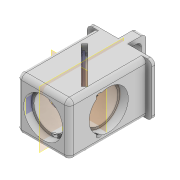
# Autodesk Inventor part: 30_Cube_Insert_Filter_Revolver_Filter_base_single_v3
Saved by Autodesk Inventor 2022 (Build 260153000, 153)
## iProperties
Created: 2021-11-01
Part Number: 30_Cube_Insert_Filter_Revolver_Filter_base_single_v3
Material: Generic
Document SubType Name: Modeling
Designer: diederichbenedict
Density: 1 g/cm^3
Appearance: Default
Author: diederichbenedict
Autodesk Inventor part; units mm, degrees
ref_plane "YZ Plane" through (0, 0, 0) normal (1, 0, 0) x (0, 1, 0)
ref_plane "XZ Plane" through (0, 0, 0) normal (0, 1, 0) x (-1, 0, 0)
ref_plane "XY Plane" through (0, 0, 0) normal (0, 0, 1) x (1, 0, 0)
ref_plane "Work Plane1" through (0, -77.5771, 0) normal (0, 0, 1) x (-1, 0, 0)
sketch "Sketch1" plane through (0, -77.5771, 0) normal (0, 0, 1) x (-1, 0, 0)
  line L0 (-35.2543, -30.7885) -> (-35.2543, -38.2885) construction
  line L1 (4.5657, -30.7885) -> (-35.2543, -30.7885) construction
  line L2 (4.5657, -30.7885) -> (4.5657, 3.3115) construction
  line L3 (10.4457, 3.3115) -> (4.5657, 3.3115) construction
  line L4 (10.4457, -38.2885) -> (10.4457, 3.3115) construction
  line L5 (-35.2543, -38.2885) -> (10.4457, -38.2885) construction
  line L6 (10.4457, 3.2115) -> (10.4457, 10.7115) construction
  line L7 (-29.3743, 3.2115) -> (10.4457, 3.2115) construction
  line L8 (-29.3743, 3.2115) -> (-29.3743, -30.8885) construction
  line L9 (-35.2543, -30.8885) -> (-29.3743, -30.8885) construction
  line L10 (-35.2543, 10.7115) -> (-35.2543, -30.8885) construction
  line L11 (10.4457, 10.7115) -> (-35.2543, 10.7115) construction
  line L12 (4.5657, 3.3115) -> (-29.3743, 3.3115) construction
  line L13 (-29.3743, 3.3115) -> (-29.3743, -30.8885) construction
  line L14 (-29.3743, -30.8885) -> (4.5657, -30.8885) construction
  line L15 (4.5657, -30.8885) -> (4.5657, 3.3115) construction
  line L16 (-29.3543, -30.7385) -> (4.5457, -30.7385)
  line L17 (4.5457, -30.7385) -> (4.5457, 3.1615)
  line L18 (4.5457, 3.1615) -> (-29.3543, 3.1615)
  line L19 (-29.3543, 3.1615) -> (-29.3543, -30.7385)
  line L20 (-29.3543, -30.7385) -> (4.5457, 3.1615) construction
  line L21 (4.5457, -30.7385) -> (-29.3543, 3.1615) construction
  line L22 (4.5457, -30.7385) -> (-29.3543, 3.1615)
  point P0 (0, -77.5771)
  point P1 (-12.4043, -13.7885)
  dimension "d0" = 33.9
  dimension "d1" = 33.9
  constraints: 22 end point, 4 parallel, 2 horizontal, 2 midpoint, 2 perpendicular
  measures "d0" distance of L18.end L17.end
  measures "d1" distance of L17.end L16.end
extrude "Extrusion1" add sketch "Sketch1" along normal mid plane 50
sketch "Sketch2" plane through (29.3543, -80.7385, 25) normal (1, 0, 0) x (0, 0, -1)
  line L0 (50, 33.9) -> (0, 33.9) projected
  line L1 (0, 0) -> (0, 33.9) projected
  line L2 (50, 0) -> (0, 0) projected
  line L3 (50, 33.9) -> (50, 0) projected
  circle A0 centre (25, 25) radius 25
  circle A1 centre (25.7081, 16.95) radius 12.75
  point P0 (25, 80.7385)
  dimension "d4" = 25.5
  constraints: 3 tangent, 2 centre point
  measures "d4" diameter of A1
extrude "Extrusion2" cut sketch "Sketch2" against normal blind 5.5 contours A1
sketch "Sketch3" plane through (29.3543, -80.7385, 25) normal (1, 0, 0) x (0, 0, -1)
  circle A0 centre (25.7081, 16.95) radius 12.75 projected
  circle A1 centre (25.7081, 16.95) radius 11.5
  point P0 (25, 80.7385)
  dimension "d7" = 23
  constraints: 1 centre point, 1 coincident
  measures "d7" diameter of A1
extrude "Extrusion3" cut sketch "Sketch3" against normal through all contours A1
sketch "Sketch4" plane through (0, -77.5771, 25) normal (0, 0, 1) x (1, 0, 0)
  line L0 (-4.5457, 30.7385) -> (-4.5457, -3.1615) projected
  line L1 (-4.5457, -3.1615) -> (29.3543, -3.1615) projected
  line L2 (29.3543, -3.1615) -> (29.3543, 30.7385) projected
  line L3 (29.3543, 30.7385) -> (-4.5457, 30.7385) projected
  circle A0 centre (12.4043, 13.7885) radius 12.75
  point P0 (0, 77.5771)
  dimension "d10" = 25.5
  constraints: 1 centre point
  measures "d10" diameter of A0
extrude "Extrusion4" cut sketch "Sketch4" against normal blind 5 contours A0
sketch "Sketch5" plane through (0, -77.5771, 25) normal (0, 0, 1) x (1, 0, 0)
  circle A0 centre (12.4043, 13.7885) radius 12.75 projected
  circle A1 centre (12.4043, 13.7885) radius 11
  point P0 (0, 77.5771)
  dimension "d13" = 22
  constraints: 1 centre point, 1 coincident
  measures "d13" diameter of A1
extrude "Extrusion5" cut sketch "Sketch5" against normal up to surface contours A1 round surface about axis through (29.3543, -63.7885, -0.7081) along (-1, 0, 0) radius 11.5 far side no
sketch "Sketch6" plane through (-4.5457, -80.7385, 25) normal (0, -1, 0) x (1, 0, 0)
  line L0 (16.95, -60.29) -> (16.95, 9.29)
  line L1 (-17.84, -25.5) -> (51.74, -25.5)
  line L2 (2.1008, -40.3492) -> (31.7992, -10.6508)
  line L3 (31.7992, -10.6508) -> (32.7185, -11.57)
  line L4 (32.7185, -11.57) -> (3.02, -41.2685)
  line L5 (3.02, -41.2685) -> (2.1008, -40.3492)
  line L6 (2.1008, -40.3492) -> (44.1008, -40.3492) construction
  circle A0 centre (3.3798, -39.9894) radius 1.3287
  circle A1 centre (31.4526, -11.9166) radius 1.3125
  point P0 (4.5457, -25)
  point P1 (16.95, -25.5)
  point P2 (31.7992, -10.6508)
  point P3 (31.7992, -10.6508)
  point P4 (30.1867, -12.2633)
  point P5 (31.106, -13.1825)
  point P6 (4.6589, -39.6296)
  point P7 (3.7396, -38.7104)
  dimension "d16" = 42
  dimension "d17" = 45
  dimension "d18" = 1.3
  constraints: 14 end point, 4 point on circle, 2 centre point, 2 horizontal, 2 midpoint, 2 parallel, 1 equal length, 1 perpendicular, 1 vertical, 4 other
  measures "d16" distance of L2.start L2.end
  measures "d17" angle of L6 L2
  measures "d18" distance of L2.end L3.end
extrude "Extrusion6" cut sketch "Sketch6" against normal blind 30
sketch "Sketch7" plane through (-4.5457, -80.7385, 25) normal (0, -1, 0) x (1, 0, 0)
  arc A0 (31.106, -13.1825) -> (30.1867, -12.2633) centre (31.4526, -11.9166) ccw projected
  line L0 (31.106, -13.1825) -> (4.6589, -39.6296) projected
  arc A1 (3.7396, -38.7104) -> (4.6589, -39.6296) centre (3.3798, -39.9894) ccw projected
  line L1 (3.7396, -38.7104) -> (30.1867, -12.2633) projected
  line L2 (33.9, -50) -> (33.9, 0) projected
  line L3 (0, 0) -> (33.9, 0) projected
  line L4 (0, -50) -> (0, 0) projected
  line L5 (33.9, -50) -> (0, -50) projected
  line L6 (28.8709, -12.8843) -> (4.8293, -36.9259)
  line L7 (4.8293, -36.9259) -> (6.9506, -39.0472)
  line L8 (6.9506, -39.0472) -> (30.9922, -15.0056)
  line L9 (30.9922, -15.0056) -> (28.8709, -12.8843)
  line L10 (28.6234, -13.1318) -> (6.7031, -39.2947) construction
  line L11 (4.5818, -37.1734) -> (30.7447, -15.2531) construction
  line L12 (28.6234, -13.1318) -> (62.6234, -13.1318) construction
  line L13 (0, -50) -> (0, 0) projected
  line L14 (4.8293, -36.9259) -> (3.2736, -38.4815)
  point P0 (4.5457, -25)
  point P1 (17.6632, -26.2132)
  dimension "d21" = 34
  dimension "d22" = 135
  dimension "d23" = 3
  dimension "d50" = 2.2
  constraints: 16 end point, 3 parallel, 2 midpoint, 2 perpendicular, 1 equal length, 1 horizontal
  measures "d21" distance of L6.start L6.end
  measures "d22" angle of L6 L12
  measures "d23" distance of L7.end L6.end
  measures "d50" distance of L14.start L14.end
extrude "Extrusion7" cut sketch "Sketch7" against normal through all contours L9 L8 L7 L0 | L0 L7 L1 L9 | L1 L7 L6 L9
sketch "Sketch8" plane through (0.2836, -80.7385, -11.9259) normal (0.7071068, 0, -0.7071068) x (-0.7071068, 0, -0.7071068)
  ellipse E0 centre (-15.8643, 16.95) end of major axis (0.3991, 16.95) minor radius 11.5 (-25.3125, 7.5897) -> (-25.3125, 26.3103) ccw projected
  line L0 (-32.8643, 5.95) -> (1.1357, 5.95)
  line L1 (1.1357, 5.95) -> (1.1357, 27.95)
  line L2 (1.1357, 27.95) -> (-32.8643, 27.95)
  line L3 (-32.8643, 27.95) -> (-32.8643, 5.95)
  line L4 (-32.8643, 5.95) -> (1.1357, 27.95) construction
  line L5 (1.1357, 5.95) -> (-32.8643, 27.95) construction
  circle A0 centre (1.1357, 27.95) radius 1.45
  circle A1 centre (1.1357, 5.95) radius 1.45
  circle A2 centre (-32.8643, 5.95) radius 1.45
  circle A3 centre (-32.8643, 27.95) radius 1.45
  point P0 (-8.2324, 80.7385)
  point P1 (0, 19.4821)
  point P2 (1.1357, 7.4)
  point P3 (-0.3143, 5.95)
  point P4 (-32.8643, 7.4)
  point P5 (-31.4143, 5.95)
  point P6 (-31.4143, 27.95)
  point P7 (-32.8643, 26.5)
  dimension "d26" = 34
  dimension "d27" = 22
  dimension "d28" = 2.9
  dimension "d29" = 2.9
  dimension "d30" = 2.9
  dimension "d31" = 2.9
  constraints: 12 end point, 4 centre point, 4 coincident, 2 midpoint, 2 parallel, 1 horizontal, 1 perpendicular, 1 other
  measures "d26" distance between parallel lines of L3 L1
  measures "d27" distance between parallel lines of L2 L0
  measures "d28" diameter of A0
  measures "d29" diameter of A1
  measures "d30" diameter of A2
  measures "d31" diameter of A3
extrude "Extrusion8" cut sketch "Sketch8" along normal through all both and the other way through all contours A2 L3 L0 | L0 L1 A1 | A0 L1 L2 | L2 L1 A0 | A3 L2 L3 picked at (-33.213, 6.8436) picked at (0.1831, 5.8343) picked at (-33.5426, 28.6283)
ref_plane "Work Plane2" through (12.3543, -80.7385, 25) normal (1, 0, 0) x (0, 0, -1)
sketch "Sketch9" plane through (12.3543, -80.7385, 25) normal (1, 0, 0) x (0, 0, -1)
  ellipse E0 centre (19.5195, 5.95) end of major axis (21.5701, 5.95) minor radius 1.45 (17.9186, 6.8562) -> (21.1283, 5.0509) ccw projected
  arc A0 (17.9186, 27.0438) -> (17.9186, 6.8562) centre (25.7081, 16.95) ccw projected
  ellipse E1 centre (19.5195, 27.95) end of major axis (21.5701, 27.95) minor radius 1.45 (21.1283, 28.8491) -> (17.9186, 27.0438) ccw projected
  arc A1 (21.1283, 5.0509) -> (21.1283, 28.8491) centre (25.7081, 16.95) ccw projected
  line L0 (50, 33.9) -> (0, 33.9) projected
  line L1 (0, 0) -> (0, 33.9) projected
  line L2 (50, 0) -> (0, 0) projected
  line L3 (50, 33.9) -> (50, 0) projected
  line L4 (50, 33.9) -> (50, 0) projected
  line L5 (50, 0) -> (64, 0)
  line L6 (64, 0) -> (64, 33.9)
  line L7 (64, 33.9) -> (50, 33.9)
  line L8 (50, 33.9) -> (50, 0)
  line L9 (61, 30.9) -> (61, 3)
  line L10 (61, 3) -> (53, 3)
  line L11 (53, 3) -> (53, 30.9)
  line L12 (53, 30.9) -> (61, 30.9)
  point P0 (25, 80.7385)
  point P1 (50, 33.9)
  dimension "d35" = 14
  dimension "d36" = 3
  constraints: 16 end point, 4 parallel, 2 perpendicular, 1 horizontal, 5 other
  measures "d35" distance of L7.end L6.end
  measures "d36" distance between parallel lines of L6 L9
extrude "Extrusion9" add sketch "Sketch9" along normal mid plane 6 contours L7 L6 L5 L3
fillet "Fillet1" radius 3 14 edges at (12.3543, -80.7385, -39) (12.3543, -46.8385, -39) (12.3543, -49.8385, -28) (12.3543, -77.7385, -36) (12.3543, -77.7385, -28) (12.3543, -49.8385, -36) (12.4043, -80.7385, 25) (12.4043, -46.8385, 25) (29.3543, -63.7885, 25) (-4.5457, -63.7885, 25) (-4.5457, -80.7385, 0) (29.3543, -80.7385, 0) (29.3543, -46.8385, 0) (-4.5457, -46.8385, 0)
sketch "Sketch10" plane through (0, -77.5771, -25) normal (0, 0, -1) x (-1, 0, 0)
  arc A0 (4.5457, 27.7385) -> (1.5457, 30.7385) centre (1.5457, 27.7385) ccw projected
  line L0 (1.5457, 30.7385) -> (-9.3543, 30.7385) projected
  line L1 (-9.3543, 30.7385) -> (-9.3543, -3.1615) projected
  line L2 (-9.3543, -3.1615) -> (1.5457, -3.1615) projected
  arc A1 (1.5457, -3.1615) -> (4.5457, -0.1615) centre (1.5457, -0.1615) ccw projected
  line L3 (4.5457, -0.1615) -> (4.5457, 27.7385) projected
  arc A2 (-26.3543, 30.7385) -> (-29.3543, 27.7385) centre (-26.3543, 27.7385) ccw projected
  line L4 (-29.3543, 27.7385) -> (-29.3543, -0.1615) projected
  arc A3 (-29.3543, -0.1615) -> (-26.3543, -3.1615) centre (-26.3543, -0.1615) ccw projected
  line L5 (-26.3543, -3.1615) -> (-15.3543, -3.1615) projected
  line L6 (-15.3543, -3.1615) -> (-15.3543, 30.7385) projected
  line L7 (-15.3543, 30.7385) -> (-26.3543, 30.7385) projected
  line L8 (-30.1485, -3.1615) -> (5.8515, -3.1615)
  line L9 (8.8515, -0.1615) -> (8.8515, 27.7385)
  line L10 (5.8515, 30.7385) -> (-30.1485, 30.7385)
  line L11 (-33.1485, 27.7385) -> (-33.1485, -0.1615)
  line L12 (-33.1485, -3.1615) -> (8.8515, 30.7385) construction
  line L13 (8.8515, -3.1615) -> (-33.1485, 30.7385) construction
  arc A4 (8.8515, 27.7385) -> (5.8515, 30.7385) centre (5.8515, 27.7385) ccw
  arc A5 (5.8515, -3.1615) -> (8.8515, -0.1615) centre (5.8515, -0.1615) ccw
  arc A6 (-33.1485, -0.1615) -> (-30.1485, -3.1615) centre (-30.1485, -0.1615) ccw
  arc A7 (-30.1485, 30.7385) -> (-33.1485, 27.7385) centre (-30.1485, 27.7385) ccw
  point P0 (0, 77.5771)
  point P1 (-12.1485, 13.7885)
  point P2 (-26.3543, 30.7385)
  point P3 (1.5457, -3.1615)
  dimension "d40" = 42
  dimension "d41" = 3
  constraints: 12 end point, 8 point on circle, 8 point on line, 8 tangent, 4 centre point, 3 equal radius, 2 midpoint, 2 parallel, 1 horizontal, 1 perpendicular
  measures "d40" distance of L13.end L12.end
  measures "d41" radius of A4
extrude "Extrusion10" add sketch "Sketch10" along normal blind 2 contours L3 A1 L2 L1 L0 A0 | A0 L10 A4 L9 A5 L8 A1 L3 | L6 L5 A3 L4 A2 L7 | A2 L4 A3 L8 A6 L11 A7 L10
ref_plane "Work Plane3" through (0.5543, -77.7385, 22) normal (-1, 0, 0) x (0, 0, 1)
sketch "Sketch11" plane through (0.5543, -77.7385, 22) normal (-1, 0, 0) x (0, 0, 1)
  circle A0 centre (-22.7081, 13.95) radius 12.65
  point P0 (-22, 77.7385)
  dimension "d45" = 25.3
  constraints: 1 centre point, 1 coincident
  measures "d45" diameter of A0
extrude "Extrusion11" cut sketch "Sketch11" along normal up to surface (5.1 mm away)
ref_plane "Work Plane4" through (24.3543, -77.7385, 22) normal (1, 0, 0) x (0, 0, -1)
body "Solid1"
